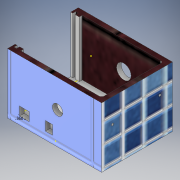
# Autodesk Inventor part: Boxpt1
Saved by Autodesk Inventor 2018.2 (Build 222227000, 227)
## iProperties
Created: 2018-04-06
Part Number: Boxpt1
Material: Generic
Document SubType Name: Modeling
Designer: MIABo
Density: 1 g/cm^3
Appearance: Default
Author: MIABo
## iProperties of the stored document Boxpt1_3DPrint.ipt
Created: 2018-04-09
Part Number: Boxpt1_3DPrint
Material: Generic
Document SubType Name: Modeling
Designer: MIABo
Density: 1 g/cm^3
Appearance: Default
Author: MIABo
Autodesk Inventor part; units mm, degrees
ref_plane "YZ Plane" through (0, 0, 0) normal (1, 0, 0) x (0, 1, 0)
ref_plane "XZ Plane" through (0, 0, 0) normal (0, 1, 0) x (-1, 0, 0)
ref_plane "XY Plane" through (0, 0, 0) normal (0, 0, 1) x (1, 0, 0)
sketch "Sketch1" plane through (0, 0, 0) normal (0, 1, 0) x (-1, 0, 0)
  line L0 (50.8, 37.719) -> (-50.8, 37.719)
  line L1 (-50.8, 37.719) -> (-50.8, -37.719)
  line L2 (-50.8, -37.719) -> (50.8, -37.719)
  line L3 (50.8, -37.719) -> (50.8, 37.719)
  line L4 (50.8, 37.719) -> (-50.8, -37.719) construction
  line L5 (-50.8, 37.719) -> (50.8, -37.719) construction
  line L6 (56.515, 43.434) -> (-56.515, 43.434)
  line L7 (-56.515, 43.434) -> (-56.515, -43.434)
  line L8 (-56.515, -43.434) -> (56.515, -43.434)
  line L9 (56.515, -43.434) -> (56.515, 43.434)
  line L10 (56.515, 43.434) -> (-56.515, -43.434) construction
  line L11 (-56.515, 43.434) -> (56.515, -43.434) construction
  point P0 (0, 0)
  dimension "d0" = 101.6
  dimension "d1" = 75.438
  dimension "d2" = 113.03
  dimension "d3" = 86.868
  constraints: 24 end point, 4 midpoint, 4 parallel, 2 horizontal, 2 perpendicular
  measures "d0" distance of L2.end L1.end
  measures "d1" distance of L1.end L0.end
  measures "d2" distance of L8.end L7.end
  measures "d3" distance of L7.end L6.end
extrude "Extrusion1" add sketch "Sketch1" along normal blind 68.58
sketch "Sketch2" plane through (0, 0, 0) normal (0, -1, 0) x (1, 0, 0)
  line L0 (-50.8, 37.719) -> (50.8, 37.719) projected
  line L1 (-50.8, 37.719) -> (-41.656, 37.719)
  line L2 (-50.8, 37.719) -> (-50.8, -37.719) projected
  line L3 (-41.656, 37.719) -> (-50.8, 37.719)
  line L4 (-50.8, 37.719) -> (-41.656, 37.719)
  point P0 (0, 0)
  dimension "d6" = 9.144
  constraints: 6 end point, 1 collinear, 1 perpendicular, 1 point on line
  measures "d6" distance of L0.start L1.end
sketch "Sketch3" plane through (-56.515, 0, 43.434) normal (0, 0, 1) x (1, 0, 0)
  line L0 (12.3133, 0) -> (12.3133, 10.668)
  line L1 (12.3133, 10.668) -> (12.3133, 14.986)
  line L2 (12.3133, 14.986) -> (24.3021, 14.986)
  line L3 (24.3021, 14.986) -> (24.3021, 4.318)
  line L4 (24.3021, 4.318) -> (12.3133, 4.318)
  line L5 (0, 0) -> (113.03, 0) projected
  line L6 (24.3021, 4.318) -> (44.2157, 4.318)
  line L7 (44.2157, 4.318) -> (44.2157, 15.494)
  line L8 (44.2157, 15.494) -> (52.9279, 15.494)
  line L9 (52.9279, 15.494) -> (52.9279, 4.318)
  line L10 (52.9279, 4.318) -> (44.2157, 4.318)
  point P0 (56.515, 0)
  dimension "d7" = 10.668
  dimension "d8" = 4.318
  dimension "d9" = 11.9888
  dimension "d10" = 10.668
  dimension "d11" = 19.9136
  dimension "d12" = 11.176
  dimension "d13" = 8.7122
  constraints: 20 end point, 7 perpendicular, 4 point on line, 1 horizontal, 1 vertical
  measures "d7" distance of L0.start L0.end
  measures "d8" distance of L0.end L1.end
  measures "d9" distance of L1.end L2.end
  measures "d10" distance of L2.end L3.end
  measures "d11" distance of L3.end L6.end
  measures "d12" distance of L6.end L7.end
  measures "d13" distance of L7.end L8.end
extrude "Extrusion2" cut sketch "Sketch3" against normal blind 68.58
sketch "Sketch4" plane through (50.8, 0, 37.719) normal (-1, 0, 0) x (0, 0, 1)
  line L0 (0, 0) -> (-75.438, 0) projected
  line L1 (-75.438, 0) -> (-34.29, 0)
  line L2 (-34.29, 0) -> (-75.438, 0)
  line L3 (-75.438, 0) -> (-75.438, 68.58) projected
  line L4 (-75.438, 0) -> (-75.438, 41.148)
  line L5 (-75.438, 41.148) -> (-65.532, 41.148)
  line L6 (-65.532, 41.148) -> (-75.438, 41.148)
  line L7 (0, 0) -> (0, 68.58) projected
  line L8 (0, 68.58) -> (0, 39.116)
  line L9 (0, 39.116) -> (0, 46.736)
  line L10 (0, 46.736) -> (0, 39.116)
  line L11 (0, 39.116) -> (-7.62, 39.116)
  line L12 (-7.62, 39.116) -> (0, 39.116)
  circle A0 centre (-7.62, 39.116) radius 1.397
  circle A1 centre (-65.532, 41.148) radius 1.397
  point P0 (-37.719, 0)
  dimension "d16" = 41.148
  dimension "d17" = 41.148
  dimension "d18" = 9.906
  dimension "d19" = 29.464
  dimension "d20" = 7.62
  dimension "d21" = 7.62
  dimension "d22" = 2.794
  dimension "d23" = 2.794
  constraints: 20 end point, 4 point on line, 3 collinear, 3 perpendicular, 2 centre point, 2 coincident
  measures "d16" distance of L0.end L1.end
  measures "d17" distance of L0.end L4.end
  measures "d18" distance of L4.end L5.end
  measures "d19" distance of L7.end L8.end
  measures "d20" distance of L8.end L9.end
  measures "d21" distance of L8.end L11.end
  measures "d22" diameter of A0
  measures "d23" diameter of A1
extrude "Extrusion3" cut sketch "Sketch4" against normal blind 68.58
sketch "Sketch5" plane through (-56.515, 0, 43.434) normal (0, 0, 1) x (1, 0, 0)
  point P0 (56.515, 0)
sketch "Sketch6" plane through (-56.515, 0, 43.434) normal (0, 0, 1) x (1, 0, 0)
  line L0 (0, 0) -> (0, 68.58) projected
  line L1 (113.03, 0) -> (113.03, 68.58) projected
  line L2 (0, 68.58) -> (113.03, 0)
  line L3 (113.03, 0) -> (0, 68.58)
  line L4 (0, 68.58) -> (113.03, 68.58) projected
  line L5 (113.03, 68.58) -> (5.08, 0)
  line L6 (5.08, 0) -> (113.03, 68.58)
  circle A0 centre (59.055, 34.29) radius 6.35
  point P0 (56.515, 0)
  dimension "d26" = 12.7
  constraints: 8 end point, 2 collinear, 1 centre point, 1 midpoint
  measures "d26" diameter of A0
extrude "Extrusion4" cut sketch "Sketch6" against normal blind 109.855 contours A0 L5 L2 | L2 L5 A0 | L5 L2 A0 | L5 A0 L2
sketch "Sketch7" plane through (0, 0, 0) normal (0, -1, 0) x (1, 0, 0)
  line L0 (-56.515, 43.434) -> (56.515, 43.434) projected
  line L1 (56.515, 43.434) -> (56.515, -43.434) projected
  line L2 (-56.515, 43.434) -> (56.515, 43.434)
  line L3 (56.515, 43.434) -> (56.515, -43.434)
  line L4 (56.515, -43.434) -> (-56.515, -43.434)
  line L5 (-56.515, -43.434) -> (-56.515, 43.434)
  point P0 (0, 0)
  constraints: 8 end point, 2 parallel, 1 horizontal, 1 perpendicular
extrude "Extrusion5" add sketch "Sketch7" along normal blind 5.08
sketch "Sketch9" plane through (0, 68.58, 0) normal (0, 1, 0) x (1, 0, 0)
  point P0 (0, 0)
sketch "Sketch10" plane through (50.8, 68.58, -37.719) normal (-1, 0, 0) x (0, 0, 1)
  circle A0 centre (67.818, -29.464) radius 1.397 projected
  circle A1 centre (67.818, -29.464) radius 3.302
  circle A2 centre (9.906, -27.432) radius 1.397 projected
  circle A3 centre (9.906, -27.432) radius 3.302
  point P0 (37.719, -68.58)
  dimension "d36" = 6.604
  dimension "d37" = 6.604
  constraints: 2 centre point, 2 coincident
  measures "d36" diameter of A1
  measures "d37" diameter of A3
extrude "Extrusion7" add sketch "Sketch10" along normal blind 12.7
sketch "Sketch11" plane through (-56.515, 68.58, -43.434) normal (-1, 0, 0) x (0, 0, 1)
  line L0 (5.715, -68.58) -> (5.715, 0) projected
  line L1 (81.153, -68.58) -> (81.153, 0) projected
  line L2 (5.715, 0) -> (81.153, 0)
  line L3 (81.153, 0) -> (81.153, -68.58)
  line L4 (81.153, -68.58) -> (5.715, -68.58)
  line L5 (5.715, -68.58) -> (5.715, 0)
  point P0 (43.434, -68.58)
  constraints: 8 end point, 2 parallel, 1 horizontal, 1 perpendicular
extrude "Extrusion8" cut sketch "Sketch11" against normal blind 12.7
fillet "Fillet2" radius 3.175 3 edges at (50.8, 34.29, -37.719) (50.8, 0, 0) (50.8, 34.29, 37.719)
sketch "Sketch12" plane through (56.515, 68.58, -43.434) normal (0, 0, -1) x (-1, 0, 0)
  circle A0 centre (53.975, -34.29) radius 4.445
  circle A1 centre (53.975, -34.29) radius 8.89
  circle A2 centre (53.975, -34.29) radius 6.35 projected
  point P0 (56.515, -68.58)
  dimension "d43" = 8.89
  dimension "d44" = 17.78
  constraints: 2 centre point, 1 coincident, 1 concentric
  measures "d43" diameter of A0
  measures "d44" diameter of A1
extrude "Extrusion9" cut sketch "Sketch12" against normal blind 12.7 contours A1
sketch "Sketch13" plane through (0, 0, 0) normal (0, 1, 0) x (1, 0, 0)
  line L0 (-56.515, 37.719) -> (47.625, 37.719) projected
  line L1 (-50.7189, 37.719) -> (-49.9627, 37.719)
  line L2 (-49.9627, 37.719) -> (-49.9627, 36.449)
  line L3 (-49.9627, 36.449) -> (-50.7189, 36.449)
  line L4 (-50.7189, 36.449) -> (-50.7189, 37.719)
  line L5 (-56.515, -37.719) -> (47.625, -37.719) projected
  line L6 (-50.7189, -37.719) -> (-49.9627, -37.719)
  line L7 (-49.9627, -37.719) -> (-49.9627, -36.449)
  line L8 (-49.9627, -36.449) -> (-50.7189, -36.449)
  line L9 (-50.7189, -36.449) -> (-50.7189, -37.719)
  point P0 (0, 0)
  dimension "d47" = 1.27
  dimension "d48" = 1.27
  constraints: 16 end point, 4 parallel, 2 horizontal, 2 perpendicular, 2 point on line
  measures "d47" distance of L1.end L2.end
  measures "d48" distance of L7.end L6.end
extrude "Extrusion10" add sketch "Sketch13" along normal blind 68.58
sketch "Sketch14" plane through (-56.515, -5.08, -43.434) normal (-1, 0, 0) x (0, 0, 1)
  point P0 (43.434, 5.08)
sketch "Sketch15" plane through (-56.515, -5.08, -43.434) normal (-1, 0, 0) x (0, 0, 1)
  line L0 (0, 73.66) -> (5.715, 73.66) projected
  line L1 (86.868, 0) -> (0, 0) projected
  line L2 (0, 73.66) -> (4.5789, 73.66)
  line L3 (4.5789, 73.66) -> (4.5789, 0)
  line L4 (4.5789, 0) -> (0, 0)
  line L5 (0, 0) -> (0, 73.66)
  line L6 (81.153, 73.66) -> (86.868, 73.66) projected
  line L7 (86.868, 73.66) -> (77.4615, 73.66)
  line L8 (77.4615, 73.66) -> (77.4615, 0)
  line L9 (77.4615, 0) -> (86.868, 0)
  line L10 (86.868, 0) -> (86.868, 73.66)
  line L11 (4.5789, 0) -> (77.4615, 0)
  line L12 (77.4615, 0) -> (77.4615, 5.08)
  line L13 (77.4615, 5.08) -> (4.5789, 5.08)
  line L14 (4.5789, 5.08) -> (4.5789, 0)
  point P0 (43.434, 5.08)
  constraints: 24 end point, 6 parallel, 3 horizontal, 3 perpendicular, 3 point on line
extrude "Extrusion11" add sketch "Sketch15" along normal blind 0.762
sketch "Sketch16" plane through (-57.277, -5.08, -43.434) normal (-1, 0, 0) x (0, 0, 1)
  line L0 (0, 0) -> (86.868, 0) projected
  line L1 (0, 73.66) -> (4.5551, 73.66)
  line L2 (4.5551, 73.66) -> (4.5551, 0)
  line L3 (4.5551, 0) -> (0, 0)
  line L4 (0, 0) -> (0, 73.66)
  line L5 (86.868, 73.66) -> (77.4615, 73.66) projected
  line L6 (86.868, 0) -> (86.868, 73.66) projected
  line L7 (77.4615, 73.66) -> (86.868, 73.66)
  line L8 (86.868, 73.66) -> (86.868, 0)
  line L9 (86.868, 0) -> (77.4615, 0)
  line L10 (77.4615, 0) -> (77.4615, 73.66)
  line L11 (79.883, 5.08) -> (81.153, 5.08) projected
  line L12 (79.883, 5.08) -> (4.5551, 5.08)
  line L13 (4.5551, 5.08) -> (4.5551, 0)
  line L14 (4.5551, 0) -> (79.883, 0)
  line L15 (79.883, 0) -> (79.883, 5.08)
  point P0 (43.434, 5.08)
  constraints: 24 end point, 6 parallel, 3 horizontal, 3 perpendicular, 1 point on line
extrude "Extrusion12" add sketch "Sketch16" along normal blind 1.5875
sketch "Sketch17" plane through (-49.9627, 0, 36.449) normal (1, 0, 0) x (0, 0, -1)
  line L0 (-1.27, 68.58) -> (0, 68.58) projected
  line L1 (0, 68.58) -> (-1.27, 68.58)
  line L2 (-1.27, 68.58) -> (-1.27, 0)
  line L3 (-1.27, 0) -> (0, 0)
  line L4 (0, 0) -> (0, 68.58)
  line L5 (74.168, 0) -> (72.898, 0) projected
  line L6 (72.898, 0) -> (72.898, 68.58) projected
  line L7 (74.168, 0) -> (72.898, 0)
  line L8 (72.898, 0) -> (72.898, 68.58)
  line L9 (72.898, 68.58) -> (74.168, 68.58)
  line L10 (74.168, 68.58) -> (74.168, 0)
  point P0 (36.449, 0)
  constraints: 16 end point, 4 parallel, 2 horizontal, 2 perpendicular
extrude "Extrusion13" add sketch "Sketch17" along normal blind 1.5875
sketch "Sketch18" plane through (-50.7189, 0, -36.449) normal (-1, 0, 0) x (0, 0, 1)
  point P0 (36.449, 0)
sketch "Sketch19" plane through (-57.277, 0, -38.8789) normal (0, 0, 1) x (1, 0, 0)
  line L0 (-1.5875, 68.58) -> (-1.5875, -5.08) projected
  line L1 (-1.5875, 68.58) -> (0.8838, 68.58)
  line L2 (0.8838, 68.58) -> (0.8838, 0)
  line L3 (0.8838, 0) -> (-1.5875, 0)
  line L4 (-1.5875, 0) -> (-1.5875, 68.58)
  point P0 (57.277, 0)
  constraints: 8 end point, 2 parallel, 1 horizontal, 1 perpendicular
extrude "Extrusion14" add sketch "Sketch19" along normal blind 4.826
sketch "Sketch20" plane through (0, 68.58, 0) normal (0, 1, 0) x (1, 0, 0)
  point P0 (0, 0)
sketch "Sketch21" plane through (0, 0, 0) normal (0, 1, 0) x (1, 0, 0)
  line L0 (-56.515, -37.719) -> (-56.515, -34.0275) projected
  line L1 (-56.515, -37.719) -> (-53.34, -37.719)
  line L2 (-50.7189, -37.719) -> (-56.515, -37.719) projected
  line L3 (-53.34, -37.719) -> (-56.515, -37.719)
  line L4 (-56.3932, 37.719) -> (-56.3932, 34.0529) projected
  line L5 (-56.3932, 37.719) -> (-53.2182, 37.719)
  line L6 (-56.3932, 37.719) -> (-50.7189, 37.719) projected
  line L7 (-53.2182, 37.719) -> (-56.3932, 37.719)
  line L8 (-53.2182, 37.719) -> (-48.4756, 37.719)
  line L9 (-48.4756, 37.719) -> (-48.4756, 34.0529)
  line L10 (-48.4756, 34.0529) -> (-53.2182, 34.0529)
  line L11 (-53.2182, 34.0529) -> (-53.2182, 37.719)
  line L12 (-53.34, -37.719) -> (-48.4756, -37.719)
  line L13 (-48.4756, -37.719) -> (-48.4756, -34.0275)
  line L14 (-48.4756, -34.0275) -> (-53.34, -34.0275)
  line L15 (-53.34, -34.0275) -> (-53.34, -37.719)
  point P0 (0, 0)
  dimension "d59" = 3.175
  dimension "d60" = 3.175
  constraints: 24 end point, 4 parallel, 3 point on line, 2 collinear, 2 horizontal, 2 perpendicular
  measures "d59" distance of L0.start L1.end
  measures "d60" distance of L4.start L5.end
extrude "Extrusion15" add sketch "Sketch21" along normal blind 68.58
body "Solid1"
